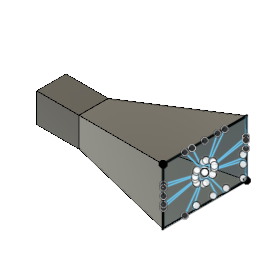
ion thruster-4 v1 (Autodesk Fusion 360 design; units mm, degrees)
Autodesk Fusion 360 part; units mm, degrees
sketch "Skizze7" plane through (0, 0, 0) normal (1, 0, 0) x (0, 1, 0)
  line L0 (-53, 53) -> (53, 53)
  line L1 (53, 53) -> (53, -53)
  line L2 (53, -53) -> (-53, -53)
  line L3 (-53, -53) -> (-53, 53)
  line L4 (-53, 53) -> (53, -53) construction
  line L5 (53, 53) -> (-53, -53) construction
  dimension "d31" = 106
  dimension "d32" = 106
  constraint horizontal L0
  constraint perpendicular L0 L1
  constraint parallel L0 L2
  constraint parallel L1 L3
  constraint coincident L4 origin
  constraint coincident L5 origin
  measures "d31" distance of L1.end L2.end
  measures "d32" distance of L0.end L1.end
extrude "Extrusion4" add sketch "Skizze7" against normal blind 153 makes body 1
sketch "Skizze8" plane through (0, 0, 0) normal (1, 0, 0) x (0, 1, 0)
  line L0 (50, -50) -> (-50, -50)
  line L1 (-50, -50) -> (-50, 50)
  line L2 (-50, 50) -> (50, 50)
  line L3 (50, 50) -> (50, -50)
  line L4 (50, -50) -> (-50, 50) construction
  line L5 (-50, -50) -> (50, 50) construction
  dimension "d35" = 100
  dimension "d36" = 100
  constraint horizontal L0
  constraint perpendicular L0 L1
  constraint parallel L0 L2
  constraint parallel L1 L3
  constraint coincident L4 origin
  constraint coincident L5 origin
  measures "d35" distance of L1.end L2.end
  measures "d36" distance of L0.end L1.end
extrude "Extrusion5" cut sketch "Skizze8" against normal blind 150 bodies 1
sketch "Skizze9" plane through (-153, 0, 0) normal (-1, 0, 0) x (0, -1, 0)
  line L0 (-53, -53) -> (53, -53)
  line L1 (53, -53) -> (53, 53)
  line L2 (53, 53) -> (-53, 53)
  line L3 (-53, 53) -> (-53, -53)
  line L4 (53, 53) -> (-53, 53)
  line L5 (-53, 53) -> (-53, -53)
  line L6 (-53, -53) -> (53, -53)
  line L7 (53, -53) -> (53, 53)
  circle A0 centre (0, 0) radius 9
  line L8 (-6.1659, -16.9405) -> (-14.5398, -39.9479)
  line L9 (-16.2488, -5.9141) -> (-39.9479, -14.5398)
  line L10 (-16.9405, 6.1659) -> (-39.9479, 14.5398)
  line L11 (-5.9141, 16.2488) -> (-15.0283, 41.2899)
  line L12 (5.9141, 16.2488) -> (15.0283, 41.2899)
  line L13 (16.2488, 5.9141) -> (41.2899, 15.0283)
  line L14 (16.2488, -5.9141) -> (41.2899, -15.0283)
  line L15 (6.1659, -16.9405) -> (14.5398, -39.9479)
  line L16 (-7.6189, -16.3387) -> (-20.7673, -44.5357)
  line L17 (16.3387, -7.6189) -> (44.5357, -20.7673)
  line L18 (7.6189, -16.3387) -> (20.7673, -44.5357)
  line L19 (7.3078, 15.6715) -> (21.0366, 45.1131)
  line L20 (15.6715, 7.3078) -> (45.1131, 21.0366)
  line L21 (-15.6715, 7.3078) -> (-45.1131, 21.0366)
  line L22 (-7.3078, 15.6715) -> (-21.0366, 45.1131)
  line L23 (-42, -48) -> (-26.2052, -48)
  line L24 (-48, 8.9017) -> (-48, -8.9017)
  line L25 (-48, -26.2052) -> (-48, -42)
  line L26 (-8.9017, -48) -> (8.9017, -48)
  line L27 (26.2052, -48) -> (42, -48)
  line L28 (48, -42) -> (48, -26.2052)
  line L29 (48, -10.3298) -> (48, 10.3298)
  line L30 (48, 25.5681) -> (48, 43)
  line L31 (43, 48) -> (25.5681, 48)
  line L32 (-16.3387, -7.6189) -> (-44.5357, -20.7673)
  arc A1 (8.9335, -9.4441) -> (9.4441, -8.9335) centre (0, 0) ccw
  arc A2 (12.9703, -0.8779) -> (12.9703, 0.8779) centre (0, 0) ccw
  arc A3 (9.7922, 8.5506) -> (8.5506, 9.7922) centre (0, 0) ccw
  arc A4 (0.8779, 12.9703) -> (-0.8779, 12.9703) centre (0, 0) ccw
  arc A5 (-8.5506, 9.7922) -> (-9.7922, 8.5506) centre (0, 0) ccw
  arc A6 (-12.995, 0.3611) -> (-12.9703, -0.8779) centre (0, 0) ccw
  arc A7 (-9.4441, -8.9335) -> (-8.9335, -9.4441) centre (0, 0) ccw
  arc A8 (-0.3611, -12.995) -> (0.3611, -12.995) centre (0, 0) ccw
  arc A9 (8.9335, -9.4441) -> (7.6189, -16.3387) centre (13.0567, -13.803) ccw
  arc A10 (16.3387, -7.6189) -> (9.4441, -8.9335) centre (13.803, -13.0567) ccw
  arc A11 (48, -26.2052) -> (44.5357, -20.7673) centre (42, -26.2052) ccw
  arc A12 (20.7673, -44.5357) -> (26.2052, -48) centre (26.2052, -42) ccw
  arc A13 (42, -48) -> (48, -42) centre (42, -42) ccw
  arc A14 (6.1659, -16.9405) -> (0.3611, -12.995) centre (0.5277, -18.9927) ccw
  arc A15 (-0.3611, -12.995) -> (-6.1659, -16.9405) centre (-0.5277, -18.9927) ccw
  arc A16 (-14.5398, -39.9479) -> (-8.9017, -48) centre (-8.9017, -42) ccw
  arc A17 (8.9017, -48) -> (14.5398, -39.9479) centre (8.9017, -42) ccw
  arc A18 (-7.6189, -16.3387) -> (-8.9335, -9.4441) centre (-13.0567, -13.803) ccw
  arc A19 (-9.4441, -8.9335) -> (-16.3387, -7.6189) centre (-13.803, -13.0567) ccw
  arc A20 (-44.5357, -20.7673) -> (-48, -26.2052) centre (-42, -26.2052) ccw
  arc A21 (-48, -42) -> (-42, -48) centre (-42, -42) ccw
  arc A22 (-26.2052, -48) -> (-20.7673, -44.5357) centre (-26.2052, -42) ccw
  arc A23 (-48, -8.9017) -> (-39.9479, -14.5398) centre (-42, -8.9017) ccw
  arc A24 (-39.9479, 14.5398) -> (-48, 8.9017) centre (-42, 8.9017) ccw
  arc A25 (-12.995, 0.3611) -> (-16.9405, 6.1659) centre (-18.9927, 0.5277) ccw
  line L33 (10.3298, 48) -> (-10.3298, 48)
  line L34 (-25.5681, 48) -> (-43, 48)
  line L35 (-48, 25.5681) -> (-48, 43)
  arc A26 (-16.2488, -5.9141) -> (-12.9703, -0.8779) centre (-17.9589, -1.2156) ccw
  arc A27 (-15.6715, 7.3078) -> (-9.7922, 8.5506) centre (-13.5584, 11.8393) ccw
  arc A28 (-8.5506, 9.7922) -> (-7.3078, 15.6715) centre (-11.8393, 13.5584) ccw
  arc A29 (0.8779, 12.9703) -> (5.9141, 16.2488) centre (1.2156, 17.9589) ccw
  arc A30 (-5.9141, 16.2488) -> (-0.8779, 12.9703) centre (-1.2156, 17.9589) ccw
  arc A31 (16.2488, 5.9141) -> (12.9703, 0.8779) centre (17.9589, 1.2156) ccw
  arc A32 (7.3078, 15.6715) -> (8.5506, 9.7922) centre (11.8393, 13.5584) ccw
  arc A33 (9.7922, 8.5506) -> (15.6715, 7.3078) centre (13.5584, 11.8393) ccw
  arc A34 (12.9703, -0.8779) -> (16.2488, -5.9141) centre (17.9589, -1.2156) ccw
  arc A35 (48, 10.3298) -> (41.2899, 15.0283) centre (43, 10.3298) ccw
  arc A36 (41.2899, -15.0283) -> (48, -10.3298) centre (43, -10.3298) ccw
  arc A37 (45.1131, 21.0366) -> (48, 25.5681) centre (43, 25.5681) ccw
  arc A38 (48, 43) -> (43, 48) centre (43, 43) ccw
  arc A39 (25.5681, 48) -> (21.0366, 45.1131) centre (25.5681, 43) ccw
  arc A40 (-48, 25.5681) -> (-45.1131, 21.0366) centre (-43, 25.5681) ccw
  arc A41 (-43, 48) -> (-48, 43) centre (-43, 43) ccw
  arc A42 (-21.0366, 45.1131) -> (-25.5681, 48) centre (-25.5681, 43) ccw
  arc A43 (-10.3298, 48) -> (-15.0283, 41.2899) centre (-10.3298, 43) ccw
  arc A44 (15.0283, 41.2899) -> (10.3298, 48) centre (10.3298, 43) ccw
  dimension "d39" = 106
  dimension "d40" = 106
  dimension "d41" = 18
  dimension "d52" = 6
  dimension "d53" = 6
  dimension "d54" = 5
  dimension "d55" = 5
  constraint horizontal L4
  constraint perpendicular L4 L5
  constraint parallel L4 L6
  constraint parallel L5 L7
  constraint coincident A0.centre A1.centre
  constraint collinear L23 L26
  constraint collinear L24 L25
  constraint collinear L26 L27
  constraint collinear L28 L29
  constraint collinear L29 L30
  constraint collinear L31 L33
  constraint concentric A0 A1
  constraint concentric A1 A2
  constraint concentric A2 A3
  constraint concentric A3 A4
  constraint concentric A4 A5
  constraint concentric A5 A6
  constraint concentric A6 A7
  constraint concentric A7 A8
  constraint tangent L18 A9
  constraint tangent A1 A9
  constraint tangent A1 A10
  constraint tangent L17 A10
  constraint tangent L28 A11
  constraint tangent L17 A11
  constraint equal A10 A11
  constraint tangent L27 A12
  constraint tangent L18 A12
  constraint equal A10 A12
  constraint tangent L28 A13
  constraint tangent L27 A13
  constraint equal A10 A13
  constraint tangent L15 A14
  constraint tangent A8 A14
  constraint equal A10 A14
  constraint tangent L8 A15
  constraint tangent A8 A15
  constraint equal A10 A15
  constraint tangent L8 A16
  constraint tangent L26 A16
  constraint equal A10 A16
  constraint tangent L15 A17
  constraint tangent L26 A17
  constraint equal A10 A17
  constraint tangent L16 A18
  constraint tangent A7 A18
  constraint equal A10 A18
  constraint tangent L32 A19
  constraint tangent A7 A19
  constraint equal A10 A19
  constraint tangent L25 A20
  constraint tangent L32 A20
  constraint equal A10 A20
  constraint tangent L23 A21
  constraint tangent L25 A21
  constraint equal A10 A21
  constraint tangent L16 A22
  constraint tangent L23 A22
  constraint equal A10 A22
  constraint tangent L9 A23
  constraint tangent L24 A23
  constraint equal A10 A23
  constraint tangent L10 A24
  constraint tangent L24 A24
  constraint equal A10 A24
  constraint tangent L10 A25
  constraint tangent A6 A25
  constraint equal A10 A25
  constraint collinear L33 L34
  constraint perpendicular L34 L35
  constraint tangent L9 A26
  constraint tangent A6 A26
  constraint tangent L21 A27
  constraint tangent A5 A27
  constraint equal A26 A27
  constraint tangent L22 A28
  constraint tangent A5 A28
  constraint equal A26 A28
  constraint tangent L12 A29
  constraint tangent A4 A29
  constraint equal A26 A29
  constraint tangent L11 A30
  constraint tangent A4 A30
  constraint equal A26 A30
  constraint tangent L13 A31
  constraint tangent A2 A31
  constraint equal A26 A31
  constraint tangent L19 A32
  constraint tangent A3 A32
  constraint equal A26 A32
  constraint tangent L20 A33
  constraint tangent A3 A33
  constraint equal A26 A33
  constraint tangent L14 A34
  constraint tangent A2 A34
  constraint equal A26 A34
  constraint tangent L13 A35
  constraint tangent L29 A35
  constraint equal A26 A35
  constraint tangent L14 A36
  constraint tangent L29 A36
  constraint equal A26 A36
  constraint tangent L20 A37
  constraint tangent L30 A37
  constraint equal A26 A37
  constraint tangent L30 A38
  constraint tangent L31 A38
  constraint equal A26 A38
  constraint tangent L19 A39
  constraint tangent L31 A39
  constraint equal A26 A39
  constraint tangent L21 A40
  constraint tangent L35 A40
  constraint equal A26 A40
  constraint tangent L34 A41
  constraint tangent L35 A41
  constraint equal A26 A41
  constraint tangent L22 A42
  constraint tangent L34 A42
  constraint equal A26 A42
  constraint tangent L11 A43
  constraint tangent L33 A43
  constraint equal A26 A43
  constraint tangent L12 A44
  constraint tangent L33 A44
  measures "d39" distance of L0.start L0.end
  measures "d40" distance of L2.end L0.start
  measures "d41" diameter of A0
  measures "d52" radius of A9
  measures "d53" radius of A10
  measures "d54" radius of A26
  measures "d55" radius of A44
extrude "Extrusion6" cut sketch "Skizze9" against normal blind 3 contours A0 | L8 L15 L26 A8 A14 A15 A16 A17 | L9 L10 L24 A6 A23 A24 A25 A26 | L11 L12 A4 L33 A29 A30 A43 A44 | L13 L14 L29 A2 A31 A34 A35 A36 | L16 L23 L25 L32 A7 A18 A19 A20 A21 A22 | L17 L18 L27 L28 A1 A9 A10 A11 A12 A13 | L19 L20 L30 L31 A3 A32 A33 A37 A38 A39 | L21 L22 A5 L34 L35 A27 A28 A40 A41 A42 bodies 1
sketch "Skizze11" plane through (0, 0, 0) normal (1, 0, 0) x (0, 1, 0)
  line L0 (10, -10) -> (-10, -10)
  line L1 (-10, -10) -> (-10, 10)
  line L2 (-10, 10) -> (10, 10)
  line L3 (10, 10) -> (10, -10)
  line L4 (10, -10) -> (-10, 10) construction
  line L5 (-10, -10) -> (10, 10) construction
  dimension "d59" = 20
  dimension "d60" = 20
  constraint horizontal L0
  constraint perpendicular L0 L1
  constraint parallel L0 L2
  constraint parallel L1 L3
  constraint coincident L4 origin
  constraint coincident L5 origin
  measures "d59" distance of L1.end L2.end
  measures "d60" distance of L0.end L1.end
sketch "Skizze12" plane through (400, 0, 0) normal (1, 0, 0) x (0, 1, 0)
  line L0 (10, 10) -> (-10, 10)
  line L1 (-10, 10) -> (-10, -10)
  line L2 (-10, -10) -> (10, -10)
  line L3 (10, -10) -> (10, 10)
  line L4 (151.5, 150) -> (-151.5, 150)
  line L5 (-151.5, 150) -> (-151.5, -53)
  line L6 (-151.5, -53) -> (151.5, -53)
  line L7 (151.5, -53) -> (151.5, 150)
  dimension "d63" = 303
  dimension "d64" = 203
  dimension "d74" = 150
  dimension "d75" = 151.5
  constraint horizontal L4
  constraint perpendicular L4 L5
  constraint parallel L4 L6
  constraint parallel L5 L7
  measures "d63" distance of L5.end L6.end
  measures "d64" distance of L4.end L5.end
  measures "d74" distance of origin L4
  measures "d75" distance of L5 origin
sketch "Skizze13" plane through (0, 0, 0) normal (1, 0, 0) x (0, 1, 0)
  line L0 (53, 53) -> (-53, 53)
  line L1 (-53, 53) -> (-53, -53)
  line L2 (-53, -53) -> (53, -53)
  line L3 (53, -53) -> (53, 53)
  line L4 (53, 53) -> (-53, -53) construction
  line L5 (-53, 53) -> (53, -53) construction
  dimension "d65" = 106
  dimension "d66" = 106
  constraint horizontal L0
  constraint perpendicular L0 L1
  constraint parallel L0 L2
  constraint parallel L1 L3
  constraint coincident L4 origin
  constraint coincident L5 origin
  measures "d65" distance of L1.end L2.end
  measures "d66" distance of L0.end L1.end
loft "Erhebung1" add profiles "Skizze13", "Skizze12" section 1 section 2 separate body makes body 2
sketch "Skizze14" plane through (400, 0, 0) normal (1, 0, 0) x (0, 1, 0)
  line L0 (151.5, -53) -> (151.5, 150)
  line L1 (151.5, 150) -> (-151.5, 150)
  line L2 (-151.5, 150) -> (-151.5, -53)
  line L3 (-151.5, -53) -> (151.5, -53)
  line L4 (148.5, 147) -> (-148.5, 147)
  line L5 (-148.5, 147) -> (-148.5, -50)
  line L6 (-148.5, -50) -> (148.5, -50)
  line L7 (148.5, -50) -> (148.5, 147)
  dimension "d67" = 297
  dimension "d68" = 197
  dimension "d72" = 147
  dimension "d73" = 148.5
  constraint horizontal L4
  constraint perpendicular L4 L5
  constraint parallel L4 L6
  constraint parallel L5 L7
  measures "d67" distance of L5.end L6.end
  measures "d68" distance of L4.end L5.end
  measures "d72" distance of origin L4
  measures "d73" distance of L5 origin
sketch "Skizze15" plane through (0, 0, 0) normal (-1, 0, 0) x (0, -1, 0)
  line L0 (-53, 53) -> (-53, -53)
  line L1 (-53, -53) -> (53, -53)
  line L2 (53, -53) -> (53, 53)
  line L3 (53, 53) -> (-53, 53)
  line L4 (-50, -50) -> (50, -50)
  line L5 (50, -50) -> (50, 50)
  line L6 (50, 50) -> (-50, 50)
  line L7 (-50, 50) -> (-50, -50)
  line L8 (-50, -50) -> (50, 50) construction
  line L9 (50, -50) -> (-50, 50) construction
  dimension "d69" = 100
  dimension "d70" = 100
  constraint horizontal L4
  constraint perpendicular L4 L5
  constraint parallel L4 L6
  constraint parallel L5 L7
  constraint coincident L8 origin
  constraint coincident L9 origin
  measures "d69" distance of L5.end L6.end
  measures "d70" distance of L4.end L5.end
loft "Erhebung2" cut profiles "Skizze15", "Skizze14" section 1 contours L4 L5 L6 L7 section 2 contours L4 L5 L6 L7 bodies 2
sketch "Skizze16" plane through (400, 0, 0) normal (1, 0, 0) x (0, 1, 0)
  line L0 (148.5, 147) -> (148.5, -50)
  line L1 (148.5, -50) -> (-148.5, -50)
  line L2 (-148.5, -50) -> (-148.5, 147)
  line L3 (-148.5, 147) -> (148.5, 147)
  line L4 (151.5, -53) -> (151.5, 150)
  line L5 (151.5, 150) -> (-151.5, 150)
  line L6 (-151.5, 150) -> (-151.5, -53)
  line L7 (-151.5, -53) -> (151.5, -53)
  line L8 (-151.5, 150) -> (151.5, 150)
  line L9 (151.5, 150) -> (151.5, -53)
  line L10 (151.5, -53) -> (-151.5, -53)
  line L11 (-151.5, -53) -> (-151.5, 150)
  line L12 (-19.7997, 75.5735) -> (-72.0363, 147)
  line L13 (0, 150) -> (0, 147)
  line L14 (-32.5699, 56.5125) -> (-148.5, 85.0322)
  line L15 (32.5699, 56.5125) -> (148.5, 85.0322)
  line L16 (19.7997, 75.5735) -> (72.0363, 147)
  line L17 (-148.5, 48.5) -> (-151.5, 48.5)
  line L18 (148.5, 48.5) -> (151.5, 48.5)
  line L19 (-32.5699, 40.4875) -> (-148.5, 11.9678)
  line L20 (-19.7997, 21.4265) -> (-72.0363, -50)
  line L21 (19.7997, 21.4265) -> (69.0401, -45.9031)
  line L22 (32.5699, 40.4875) -> (140.8889, 13.8402)
  circle A0 centre (0, 48.5) radius 20
  line L23 (45.9313, 147) -> (14.175, 78.8985)
  line L24 (-45.9313, 147) -> (-14.175, 78.8985)
  line L25 (-39.2975, -35.7738) -> (-14.175, 18.1015)
  line L26 (33.0315, 54.3243) -> (148.5, 74.6846)
  line L27 (33.0315, 42.6757) -> (136.7635, 24.3849)
  line L28 (-33.0315, 54.3243) -> (-148.5, 74.6846)
  line L29 (-33.0315, 42.6757) -> (-148.5, 22.3154)
  line L30 (-148.5, 147) -> (148.5, 147)
  line L31 (148.5, 4.1297) -> (148.5, -40)
  line L32 (138.5, -50) -> (77.1118, -50)
  line L33 (-148.5, -50) -> (-148.5, 147)
  line L34 (39.2975, -35.7738) -> (14.175, 18.1015)
  arc A1 (-21.5579, 35.8408) -> (-19.9082, 33.3783) centre (0, 48.5) ccw
  arc A2 (-19.9082, 63.6217) -> (-21.5579, 61.1592) centre (0, 48.5) ccw
  arc A3 (3.6514, 73.2319) -> (-3.6514, 73.2319) centre (0, 48.5) ccw
  arc A4 (21.5579, 61.1592) -> (19.9082, 63.6217) centre (0, 48.5) ccw
  arc A5 (-3.6514, 23.7681) -> (3.6514, 23.7681) centre (0, 48.5) ccw
  arc A6 (19.9082, 33.3783) -> (21.5579, 35.8408) centre (0, 48.5) ccw
  arc A7 (32.5699, 40.4875) -> (21.5579, 35.8408) centre (30.1811, 30.7771) ccw
  arc A8 (19.9082, 33.3783) -> (19.7997, 21.4265) centre (27.8714, 27.3297) ccw
  arc A9 (148.5, 4.1297) -> (140.8889, 13.8402) centre (138.5, 4.1297) ccw
  arc A10 (138.5, -50) -> (148.5, -40) centre (138.5, -40) ccw
  arc A11 (69.0401, -45.9031) -> (77.1118, -50) centre (77.1118, -40) ccw
  line L35 (148.5, 147) -> (148.5, 34.233)
  line L36 (-30.2344, -50) -> (30.2344, -50)
  arc A12 (30.2344, -50) -> (39.2975, -35.7738) centre (30.2344, -40) ccw
  arc A13 (-39.2975, -35.7738) -> (-30.2344, -50) centre (-30.2344, -40) ccw
  arc A14 (-3.6514, 23.7681) -> (-14.175, 18.1015) centre (-5.112, 13.8753) ccw
  arc A15 (14.175, 18.1015) -> (3.6514, 23.7681) centre (5.112, 13.8753) ccw
  arc A16 (-19.7997, 21.4265) -> (-19.9082, 33.3783) centre (-27.8714, 27.3297) ccw
  arc A17 (-21.5579, 35.8408) -> (-32.5699, 40.4875) centre (-30.1811, 30.7771) ccw
  arc A18 (-25.6132, 48.5) -> (-33.0315, 54.3243) centre (-34.7679, 44.4763) ccw
  arc A19 (-33.0315, 42.6757) -> (-25.6132, 48.5) centre (-34.7679, 52.5237) ccw
  arc A20 (-32.5699, 56.5125) -> (-21.5579, 61.1592) centre (-30.1811, 66.2229) ccw
  arc A21 (-19.9082, 63.6217) -> (-19.7997, 75.5735) centre (-27.8714, 69.6703) ccw
  arc A22 (-14.175, 78.8985) -> (-3.6514, 73.2319) centre (-5.112, 83.1247) ccw
  arc A23 (3.6514, 73.2319) -> (14.175, 78.8985) centre (5.112, 83.1247) ccw
  arc A24 (19.7997, 75.5735) -> (19.9082, 63.6217) centre (27.8714, 69.6703) ccw
  arc A25 (21.5579, 61.1592) -> (32.5699, 56.5125) centre (30.1811, 66.2229) ccw
  arc A26 (-21.5579, 35.8408) -> (-19.9082, 33.3783) centre (0, 48.5) ccw
  arc A27 (-19.9082, 63.6217) -> (-21.5579, 61.1592) centre (0, 48.5) ccw
  arc A28 (3.6514, 73.2319) -> (-3.6514, 73.2319) centre (0, 48.5) ccw
  arc A29 (33.0315, 54.3243) -> (25.6132, 48.5) centre (34.7679, 44.4763) ccw
  arc A30 (25.6132, 48.5) -> (33.0315, 42.6757) centre (34.7679, 52.5237) ccw
  arc A31 (21.5579, 61.1592) -> (19.9082, 63.6217) centre (0, 48.5) ccw
  arc A32 (19.9082, 33.3783) -> (21.5579, 35.8408) centre (0, 48.5) ccw
  arc A33 (19.9082, 33.3783) -> (21.5579, 35.8408) centre (0, 48.5) ccw
  arc A34 (-3.6514, 23.7681) -> (3.6514, 23.7681) centre (0, 48.5) ccw
  arc A35 (-21.5579, 35.8408) -> (-19.9082, 33.3783) centre (0, 48.5) ccw
  arc A36 (-19.9082, 63.6217) -> (-21.5579, 61.1592) centre (0, 48.5) ccw
  arc A37 (21.5579, 61.1592) -> (19.9082, 63.6217) centre (0, 48.5) ccw
  arc A38 (3.6514, 73.2319) -> (-3.6514, 73.2319) centre (0, 48.5) ccw
  arc A39 (136.7635, 24.3849) -> (148.5, 34.233) centre (138.5, 34.233) ccw
  dimension "d82" = 40
  dimension "d84" = 25
  dimension "d85" = 10
  dimension "d86" = 10
  dimension "d87" = 10
  dimension "d88" = 10
  dimension "d89" = 10
  dimension "d90" = 10
  constraint horizontal L8
  constraint vertical L9
  constraint horizontal L10
  constraint vertical L11
  constraint coincident L4.start L7.end
  constraint coincident L5.end L6.start
  constraint midpoint L8 L13.start
  constraint midpoint L6 L17.end
  constraint midpoint L4 L18.end
  constraint horizontal L30
  constraint vertical L31
  constraint horizontal L32
  constraint vertical L33
  constraint coincident L2.end L3.start
  constraint coincident L0 L18.start
  constraint coincident L3 L13.end
  constraint coincident L2 L17.start
  constraint coincident L0 L15.end
  constraint coincident L0 L26.end
  constraint coincident L3 L16.end
  constraint coincident L3 L23.start
  constraint coincident L3 L24.start
  constraint coincident L3 L12.end
  constraint coincident L2 L14.end
  constraint coincident L2 L28.end
  constraint coincident L2 L19.end
  constraint coincident L2 L29.end
  constraint coincident L1 L20.end
  constraint concentric A0 A5
  constraint concentric A5 A26
  constraint concentric A1 A26
  constraint concentric A2 A5
  constraint concentric A3 A5
  constraint concentric A4 A5
  constraint concentric A5 A37
  constraint concentric A5 A6
  constraint tangent L22 A7
  constraint tangent A6 A7
  constraint tangent L21 A8
  constraint tangent A6 A8
  constraint coincident L0.start L31
  constraint tangent L22 A9
  constraint tangent L31 A9
  constraint equal A8 A9
  constraint tangent L32 A10
  constraint tangent L31 A10
  constraint equal A8 A10
  constraint coincident L1.end L32
  constraint tangent L21 A11
  constraint tangent L32 A11
  constraint equal A8 A11
  constraint perpendicular L1 L35
  constraint perpendicular L35 L36
  constraint tangent L34 A12
  constraint tangent L36 A12
  constraint coincident L1.end L36
  constraint tangent L25 A13
  constraint tangent L36 A13
  constraint equal A12 A13
  constraint tangent L25 A14
  constraint tangent A5 A14
  constraint equal A12 A14
  constraint tangent L34 A15
  constraint tangent A5 A15
  constraint equal A12 A15
  constraint tangent L20 A16
  constraint tangent A1 A16
  constraint equal A12 A16
  constraint tangent L19 A17
  constraint tangent A1 A17
  constraint equal A12 A17
  constraint tangent L28 A18
  constraint tangent A18 A26
  constraint equal A12 A18
  constraint tangent L29 A19
  constraint tangent A19 A26
  constraint equal A12 A19
  constraint tangent L14 A20
  constraint tangent A2 A20
  constraint equal A12 A20
  constraint tangent L12 A21
  constraint tangent A2 A21
  constraint equal A12 A21
  constraint tangent L24 A22
  constraint tangent A3 A22
  constraint equal A12 A22
  constraint tangent L23 A23
  constraint tangent A3 A23
  constraint equal A12 A23
  constraint tangent L16 A24
  constraint tangent A4 A24
  constraint equal A12 A24
  constraint tangent L15 A25
  constraint tangent A4 A25
  constraint equal A12 A25
  constraint concentric A26 A32
  constraint concentric A27 A32
  constraint concentric A28 A32
  constraint tangent L26 A29
  constraint tangent A29 A37
  constraint tangent L27 A30
  constraint tangent A30 A37
  constraint equal A29 A30
  constraint concentric A31 A32
  constraint concentric A33 A37
  constraint concentric A34 A37
  constraint concentric A35 A37
  constraint concentric A36 A37
  constraint concentric A37 A38
  constraint tangent L35 A39
  constraint tangent L27 A39
  measures "d82" diameter of A0
  measures "d84" angle of L13 L23
  measures "d85" angle of L18 L26
  measures "d86" radius of A7
  measures "d87" radius of A8
  measures "d88" radius of A12
  measures "d89" radius of A29
  measures "d90" radius of A39
equation "d73 = ( 297 / 2 ) * 1 mm"
equation "d75 = ( 303 / 2 ) * 1 mm"
